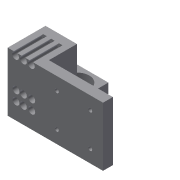
# Autodesk Inventor part: 04_Bridge_Laser_Nanomax
Saved by Autodesk Inventor 2019 (Build 230136000, 136)
## iProperties
Created: 2019-06-11
Part Number: 04_Bridge_Laser_Nanomax
Material: Generic
Document SubType Name: Modeling
Designer: diederichbenedict
Density: 1 g/cm^3
Appearance: Default
Author: diederichbenedict
Autodesk Inventor part; units mm, degrees
ref_plane "YZ Plane" through (0, 0, 0) normal (1, 0, 0) x (0, 1, 0)
ref_plane "XZ Plane" through (0, 0, 0) normal (0, 1, 0) x (-1, 0, 0)
ref_plane "XY Plane" through (0, 0, 0) normal (0, 0, 1) x (1, 0, 0)
ref_plane "Work Plane1" through (0, 0, 0) normal (0, 0, 1) x (1, 0, 0)
sketch "Sketch1" plane through (0, 0, 0) normal (0, 0, 1) x (1, 0, 0)
  arc A0 (27, -22.0618) -> (22.0618, -27) centre (24.7, -24.7) ccw construction
  line L0 (27, 0) -> (27, -22.0618) construction
  line L1 (27, 0) -> (0, 0) construction
  line L2 (0, 0) -> (0, -27) construction
  line L3 (22.0618, -27) -> (0, -27) construction
  circle A1 centre (13, -13) radius 1.65 construction
  circle A2 centre (10, -22.5) radius 1.55 construction
  circle A3 centre (10, -7.5) radius 1.55 construction
  circle A4 centre (20, -20) radius 1.05 construction
  circle A5 centre (7.5, -10) radius 1.55 construction
  circle A6 centre (22.5, -10) radius 1.55 construction
  arc A7 (22.0618, -33) -> (27, -37.9382) centre (24.7, -35.3) ccw construction
  line L4 (0, -33) -> (22.0618, -33) construction
  line L5 (0, -33) -> (0, -60) construction
  line L6 (0, -60) -> (27, -60) construction
  line L7 (27, -37.9382) -> (27, -60) construction
  circle A8 centre (13, -47) radius 1.65 construction
  circle A9 centre (10, -52.5) radius 1.55 construction
  circle A10 centre (10, -37.5) radius 1.55 construction
  circle A11 centre (20, -40) radius 1.05 construction
  circle A12 centre (7.5, -50) radius 1.55 construction
  circle A13 centre (22.5, -50) radius 1.55 construction
  arc A14 (33, -37.9382) -> (37.9382, -33) centre (35.3, -35.3) ccw construction
  line L8 (33, -60) -> (33, -37.9382) construction
  line L9 (33, -60) -> (60, -60) construction
  line L10 (60, -60) -> (60, -33) construction
  line L11 (37.9382, -33) -> (60, -33) construction
  circle A15 centre (47, -47) radius 1.65 construction
  circle A16 centre (50, -52.5) radius 1.55 construction
  circle A17 centre (50, -37.5) radius 1.55 construction
  circle A18 centre (40, -40) radius 1.05 construction
  circle A19 centre (37.5, -50) radius 1.55 construction
  circle A20 centre (52.5, -50) radius 1.55 construction
  arc A21 (37.9382, -27) -> (33, -22.0618) centre (35.3, -24.7) ccw construction
  line L12 (60, -27) -> (37.9382, -27) construction
  line L13 (60, -27) -> (60, 0) construction
  line L14 (60, 0) -> (33, 0) construction
  line L15 (33, -22.0618) -> (33, 0) construction
  circle A22 centre (47, -13) radius 1.65 construction
  circle A23 centre (50, -22.5) radius 1.55 construction
  circle A24 centre (50, -7.5) radius 1.55 construction
  circle A25 centre (40, -20) radius 1.05 construction
  circle A26 centre (37.5, -10) radius 1.55 construction
  circle A27 centre (52.5, -10) radius 1.55 construction
  line L16 (60, 0) -> (-37, 0) construction
  line L17 (-37, 0) -> (-37, -60) construction
  line L18 (-37, -60) -> (60, -60) construction
  line L19 (60, -60) -> (60, 0) construction
  line L20 (60, 0) -> (-37, 0)
  line L21 (-37, 0) -> (-37, -60)
  line L22 (-37, -60) -> (60, -60)
  line L23 (60, -60) -> (60, 0)
  line L24 (-37, 0) -> (-37, -48) projected
  constraints: 16 end point, 4 parallel, 2 horizontal, 2 perpendicular
extrude "Extrusion1" add sketch "Sketch1" along normal blind 10
sketch "Sketch2" plane through (0, 0, 0) normal (0, 0, -1) x (-1, 0, 0)
  circle A0 centre (21, -3) radius 1 projected
  circle A1 centre (28.5, -33) radius 1 projected
  circle A2 centre (12.5, -33) radius 1.0474 projected
  circle A3 centre (12.5, -43) radius 1 projected
  circle A4 centre (21, -43) radius 1 projected
  circle A5 centre (28.5, -43) radius 1 projected
  circle A6 centre (21, -33) radius 1 projected
  circle A7 centre (29, -3) radius 1 projected
  circle A8 centre (13, -3) radius 1 projected
  line L0 (37, 0) -> (5, 0) projected
  line L1 (37, 0) -> (37, -48) projected
  line L2 (5, -48) -> (37, -48) projected
  line L3 (5, 0) -> (5, -48) projected
  line L4 (37, -48) -> (5, -48)
  line L5 (5, -48) -> (5, -60)
  line L6 (5, -60) -> (37, -60)
  line L7 (37, -60) -> (37, -48)
  point P0 (0, 0)
  constraints: 8 end point, 2 parallel, 1 horizontal, 1 perpendicular
ref_plane "Work Plane2" through (-37, -48, -28.5) normal (0, 0, 1) x (1, 0, 0)
extrude "Extrusion2" add sketch "Sketch2" along normal up to surface (28.5 mm away) contours A0 | A1 | A2 | A3 | A4 | A5 | A6 | A7 | A8 | L1 L2 L3 L0 | L7 L6 L5 L2
sketch "Sketch3" plane through (0, 0, 10) normal (0, 0, 1) x (1, 0, 0)
  line L0 (0, 0) -> (0, -60) construction
  line L1 (60, 0) -> (0, 0) construction
  line L2 (60, -60) -> (60, 0) construction
  line L3 (0, -60) -> (60, -60) construction
  line L4 (27.1959, -58) -> (26.6538, -58) construction
  line L5 (27.7692, -53.6731) -> (27.1959, -58) construction
  line L6 (29.9435, -58) -> (27.7692, -53.6731) construction
  line L7 (30.0649, -58) -> (29.9435, -58) construction
  line L8 (32.2308, -53.6827) -> (30.0649, -58) construction
  line L9 (32.8053, -58) -> (32.2308, -53.6827) construction
  line L10 (33.3462, -58) -> (32.8053, -58) construction
  line L11 (32.5493, -52) -> (33.3462, -58) construction
  line L12 (32.4712, -52) -> (32.5493, -52) construction
  line L13 (30, -56.9231) -> (32.4712, -52) construction
  line L14 (27.5228, -52) -> (30, -56.9231) construction
  line L15 (27.4459, -52) -> (27.5228, -52) construction
  line L16 (26.6538, -58) -> (27.4459, -52) construction
  circle A0 centre (24.7, -24.7) radius 1.6 construction
  circle A1 centre (35.3, -24.7) radius 1.6 construction
  circle A2 centre (35.3, -35.3) radius 1.6 construction
  circle A3 centre (24.7, -35.3) radius 1.6 construction
  circle A4 centre (52.5, -50) radius 1.55 construction
  circle A5 centre (52.5, -10) radius 1.55 construction
  circle A6 centre (37.5, -50) radius 1.55 construction
  circle A7 centre (37.5, -10) radius 1.55 construction
  circle A8 centre (22.5, -50) radius 1.55 construction
  circle A9 centre (22.5, -10) radius 1.55 construction
  circle A10 centre (7.5, -50) radius 1.55 construction
  circle A11 centre (7.5, -10) radius 1.55 construction
  circle A12 centre (40, -40) radius 1.05 construction
  circle A13 centre (20, -40) radius 1.05 construction
  circle A14 centre (40, -20) radius 1.05 construction
  circle A15 centre (20, -20) radius 1.05 construction
  circle A16 centre (47, -47) radius 1.65 construction
  circle A17 centre (13, -47) radius 1.65 construction
  circle A18 centre (30, -47) radius 1.65 construction
  circle A19 centre (47, -13) radius 1.65 construction
  circle A20 centre (13, -13) radius 1.65 construction
  circle A21 centre (30, -13) radius 1.65 construction
  circle A22 centre (47, -30) radius 1.65 construction
  circle A23 centre (13, -30) radius 1.65 construction
  circle A24 centre (30, -30) radius 1.65 construction
  circle A25 centre (10, -52.5) radius 1.55 construction
  circle A26 centre (10, -37.5) radius 1.55 construction
  circle A27 centre (10, -22.5) radius 1.55 construction
  circle A28 centre (10, -7.5) radius 1.55 construction
  circle A29 centre (50, -52.5) radius 1.55 construction
  circle A30 centre (50, -37.5) radius 1.55 construction
  circle A31 centre (50, -22.5) radius 1.55 construction
  circle A32 centre (50, -7.5) radius 1.55 construction
  circle A33 centre (13, -13) radius 1.65 construction
  circle A34 centre (13, -13) radius 1.65 projected
  circle A35 centre (47, -13) radius 1.65 projected
  circle A36 centre (47, -47) radius 1.65 projected
  circle A37 centre (13, -47) radius 1.65 projected
  circle A38 centre (13, -13) radius 2
  circle A39 centre (47, -13) radius 2
  circle A40 centre (47, -47) radius 2
  circle A41 centre (13, -47) radius 2
  dimension "d6" = 4
  dimension "d7" = 4
  dimension "d8" = 4
  dimension "d9" = 4
  constraints: 4 centre point, 4 coincident
  measures "d6" diameter of A38
  measures "d7" diameter of A39
  measures "d8" diameter of A40
  measures "d9" diameter of A41
extrude "Extrusion3" cut sketch "Sketch3" against normal through all contours A34 | A35 | A36 | A37 | A38 | A39 | A40 | A41
sketch "Sketch4" plane through (0, 0, 10) normal (0, 0, 1) x (1, 0, 0)
  circle A0 centre (-21, -3) radius 1 projected
  circle A1 centre (-28.5, -33) radius 1 projected
  circle A2 centre (-12.5, -33) radius 1.0474 projected
  circle A3 centre (-12.5, -43) radius 1 projected
  circle A4 centre (-21, -43) radius 1 projected
  circle A5 centre (-28.5, -43) radius 1 projected
  circle A6 centre (-21, -33) radius 1 projected
  circle A7 centre (-29, -3) radius 1 projected
  circle A8 centre (-13, -3) radius 1 projected
  line L0 (-37, 0) -> (-5, 0) projected
  line L1 (-37, 0) -> (-37, -48) projected
  line L2 (-5, -48) -> (-37, -48) projected
  line L3 (-5, 0) -> (-5, -48) projected
  point P0 (0, 0)
hole "Hole1" at (-12.5, -43, 10) at (-21, -43, 10) at (-28.5, -43, 10) at (-28.5, -33, 10) at (-21, -33, 10) at (-12.5, -33, 10) at (-13, -3, 10) at (-21, -3, 10) at (-29, -3, 10) direction (0, 0, -1) diameter 3.5 end through all counterbore diameter 7 counterbore depth 30
sketch "Sketch5" plane through (-37, -60, 10) normal (0, -1, 0) x (1, 0, 0)
  line L0 (32, -10) -> (97, -10) projected
  line L1 (97, -10) -> (97, 0) projected
  line L2 (0, 0) -> (97, 0) projected
  line L3 (0, -38.5) -> (0, 0) projected
  line L4 (32, -38.5) -> (0, -38.5) projected
  line L5 (32, -10) -> (32, -38.5) projected
  circle A0 centre (16, -54.5) radius 2.5 construction
  line L6 (0, -70.5) -> (32, -70.5) projected
  line L7 (32, -38.5) -> (0, -38.5)
  line L8 (0, -38.5) -> (0, -70.5)
  line L9 (0, -70.5) -> (32, -70.5)
  line L10 (32, -70.5) -> (32, -38.5)
  circle A1 centre (16, -54.5) radius 12.5
  point P0 (37, -10)
  dimension "d18" = 25
  constraints: 8 end point, 2 parallel, 1 centre point, 1 coincident, 1 horizontal, 1 perpendicular
  measures "d18" diameter of A1
extrude "Extrusion4" add sketch "Sketch5" against normal blind 10 contours L10 L6 L8 L4
sketch "Sketch6" plane through (-37, -60, 10) normal (0, -1, 0) x (1, 0, 0)
  circle A0 centre (16, -54.5) radius 12.5 projected
  arc A1 (25.4152, -58.329) -> (16, -42) centre (12.4179, -54.9443) ccw
  point P0 (37, -10)
  constraints: 2 point on circle, 1 centre point, 1 vertical alignment, 1 other
body "Solid1"
